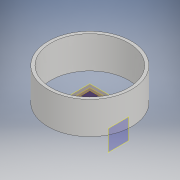
# Autodesk Inventor part: LiftMotorHousingBottom[FINAL]
Saved by Autodesk Inventor 2019 (Build 230136000, 136)
## iProperties
Created: 2018-09-19
Part Number: LiftMotorHousingBottom[FINAL]
Material: Generic
Document SubType Name: Modeling
Designer: hale985
Density: 1 g/cm^3
Appearance: Default
Author: hale985
Autodesk Inventor part; units mm, degrees
ref_plane "YZ Plane" through (0, 0, 0) normal (1, 0, 0) x (0, 1, 0)
ref_plane "XZ Plane" through (0, 0, 0) normal (0, 1, 0) x (-1, 0, 0)
ref_plane "XY Plane" through (0, 0, 0) normal (0, 0, 1) x (1, 0, 0)
ref_plane "Work Plane13" through (-2.54, 44.7855, -14.3129) normal (0, -1, 0) x (1, 0, 0)
sketch "Sketch6" plane through (-2.54, 44.7855, -14.3129) normal (0, -1, 0) x (1, 0, 0)
  line L0 (6.35, 32.4159) -> (26.9875, 32.4159) projected
  line L1 (13.4874, 32.4159) -> (13.4874, 26.0989)
  line L2 (26.9875, 32.4159) -> (26.9875, -3.9117) projected
  point P0 (2.54, 14.3129)
  dimension "d20" = 13.5001
  constraints: 2 end point, 1 point on line, 1 vertical
  measures "d20" distance between parallel lines of L2 L1
ref_plane "Work Plane14" through (-2.54, 0, 0) normal (-1, 0, 0) x (0, 0, 1)
sketch "Sketch15" plane through (-2.54, 0, 0) normal (-1, 0, 0) x (0, 0, 1)
  circle A0 centre (0, 0) radius 41.275
  circle A1 centre (0, 0) radius 44.45
  dimension "d47" = 82.55
  dimension "d48" = 88.9
  constraints: 2 centre point, 2 coincident
  measures "d47" diameter of A0
  measures "d48" diameter of A1
extrude "Extrusion11" add sketch "Sketch15" against normal blind 2.54
ref_plane "Work Plane10" through (0, 0, 0) normal (1, 0, 0) x (0, 0, -1)
sketch "Sketch16" plane through (0, 0, 0) normal (1, 0, 0) x (0, 0, -1)
  circle A0 centre (0, 0) radius 44.45
  circle A1 centre (0, 0) radius 41.275
  dimension "d51" = 82.55
  constraints: 2 centre point, 2 coincident
  measures "d51" diameter of A1
extrude "Extrusion12" add sketch "Sketch16" along normal blind 31.75
ref_plane "Work Plane9" through (-2.54, 0, 0) normal (-1, 0, 0) x (0, 0, 1)
sketch "Sketch19" plane through (-2.54, 0, 0) normal (-1, 0, 0) x (0, 0, 1)
  line L0 (4.3346, 1.4542) -> (-4.3346, 1.4542) projected
  arc A0 (-16.671, 37.7585) -> (16.671, 37.7585) centre (0, 0) ccw projected
  line L1 (-4.3346, 1.4542) -> (-41.2494, 1.4542)
  line L2 (4.3346, 1.4542) -> (41.2494, 1.4542)
  circle A1 centre (0, 0) radius 8.382
  line L3 (-4.3346, -1.4542) -> (4.3346, -1.4542)
  line L4 (4.3346, 1.4542) -> (-4.3346, 1.4542)
  line L5 (-41.2494, -1.4542) -> (41.2494, -1.4542)
  constraints: 10 end point, 4 point on circle, 2 horizontal, 1 centre point, 1 coincident, 1 parallel, 1 point on line
extrude "Extrusion14" add sketch "Sketch19" against normal blind 6.35 contours L2 A1 L5 L3 L1 L0 | L2 A0 L5 A1 | A1 L5 A0 L1
sketch "Sketch20" plane through (3.81, 0, 0) normal (1, 0, 0) x (0, 0, -1)
  line L0 (41.2494, 1.4542) -> (-41.2494, 1.4542) projected
  line L1 (-41.2494, -1.4542) -> (41.2494, -1.4542) projected
  arc A0 (-41.2494, 1.4542) -> (-41.2494, -1.4542) centre (0, 0) ccw projected
  arc A1 (41.2494, -1.4542) -> (41.2494, 1.4542) centre (0, 0) ccw projected
extrude "Extrusion15" cut sketch "Sketch20" against normal blind 6.35
ref_plane "Work Plane12" through (-2.54, 0, 0) normal (-1, 0, 0) x (0, 0, 1)
ref_plane "Work Plane11" through (3.81, 0, 0) normal (1, 0, 0) x (0, 0, -1)
body "Solid1"
